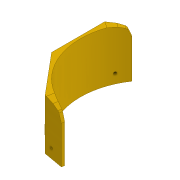
# Autodesk Inventor part: Delta Robot Siding Piece KUKA
Saved by Autodesk Inventor 2020 (Build 240168000, 168)
## iProperties
Created: 2021-04-12
Part Number: Delta Robot Siding Piece KUKA
Material: Generic
Document SubType Name: Modeling
Designer: Coy
Density: 1 g/cm^3
Appearance: Gold
Author: Coy
Autodesk Inventor part; units mm, degrees
ref_plane "YZ Plane" through (0, 0, 0) normal (1, 0, 0) x (0, 1, 0)
ref_plane "XZ Plane" through (0, 0, 0) normal (0, 1, 0) x (-1, 0, 0)
ref_plane "XY Plane" through (0, 0, 0) normal (0, 0, 1) x (1, 0, 0)
sketch "Sketch1" plane through (0, 0, 0) normal (0, 1, 0) x (-1, 0, 0)
  line L0 (68.675, -46.4884) -> (71.2969, -48.6885)
  line L1 (86.05, -31.1064) -> (71.2969, -48.6885)
  line L2 (86.05, 31.5329) -> (86.05, -31.1064)
  line L3 (45.7862, 79.5174) -> (86.05, 31.5329)
  line L4 (22.3355, 83.6524) -> (45.7862, 79.5174)
  line L5 (22.3355, 83.6524) -> (21.7555, 80.3631)
  arc A0 (68.675, -46.4884) -> (21.7555, 80.3631) centre (0, 0.2133) ccw
  constraints: 12 end point, 2 point on circle, 1 centre point
extrude "Extrusion1" add sketch "Sketch1" along normal blind 60
sketch "Sketch2" plane through (-86.05, 0, -31.1064) normal (-0.7660444, 0, -0.6427876) x (-0.6427876, 0, 0.7660444)
  circle A0 centre (-8.4518, 11) radius 1.625
  line L0 (-22.9518, 0) -> (0, 0) projected
  line L1 (-22.9518, 0) -> (-22.9518, 60) projected
  point P0 (-31.483, 0)
  dimension "d2" = 3.25
  dimension "d3" = 11
  dimension "d4" = 14.5
  constraints: 1 centre point
  measures "d2" diameter of A0
  measures "d3" distance from line of L0 A0.centre
  measures "d4" distance from line of L1 A0.centre
extrude "Extrusion2" cut sketch "Sketch2" against normal up to next
sketch "Sketch3" plane through (-22.3355, 0, 83.6524) normal (-0.1736482, 0, 0.9848078) x (0.9848078, 0, 0.1736482)
  circle A0 centre (-14.5, 11) radius 1.625
  line L0 (-23.8125, 0) -> (0, 0) projected
  line L1 (0, 0) -> (0, 60) projected
  point P0 (7.4701, 0)
  dimension "d7" = 3.25
  dimension "d8" = 11
  dimension "d9" = 14.5
  constraints: 1 centre point
  measures "d7" diameter of A0
  measures "d8" distance from line of L0 A0.centre
  measures "d9" distance from line of L1 A0.centre
extrude "Extrusion3" cut sketch "Sketch3" against normal up to next
chamfer "Chamfer5" distance 10 angle 45 2 edges at (-22.0455, 60, 82.0077) (-69.9859, 60, -47.5884)
chamfer "Chamfer6" distance 7 angle 45 2 edges at (-31.7611, 60, 79.5197) (-75.788, 60, -39.4028)
chamfer "Chamfer7" distance 5 angle 45 2 edges at (-38.4957, 60, 77.4021) (-79.5549, 60, -33.4258)
chamfer "Chamfer8" distance 5 angle 45 2 edges at (-22.0455, 50, 82.0077) (-69.9859, 50, -47.5884)
sketch "Sketch8" plane through (-86.05, 0, -31.1064) normal (-1, 0, 0) x (0, 0, 1)
  line L0 (0.07, 60.289) -> (62.7543, 60.289) construction
  line L1 (62.7543, 60.289) -> (62.7543, 0.051) construction
  line L2 (62.7543, 0.051) -> (0.07, 0.051) construction
  line L3 (0.07, 0.051) -> (0.07, 60.289) construction
  line L4 (35.582, 49.6056) -> (30.0412, 32.3549)
  line L5 (30.0412, 32.3549) -> (36.0961, 11.5056)
  line L6 (36.0961, 11.5056) -> (25.243, 11.5056)
  line L7 (25.243, 11.5056) -> (22.2156, 27.4425)
  line L8 (22.2156, 27.4425) -> (22.2156, 11.5056)
  line L9 (22.2156, 11.5056) -> (11.591, 11.5056)
  line L10 (11.591, 11.5056) -> (11.591, 49.6056)
  line L11 (11.591, 49.6056) -> (22.2156, 49.6056)
  line L12 (22.2156, 49.6056) -> (22.2156, 35.211)
  line L13 (22.2156, 35.211) -> (25.6429, 49.6056)
  line L14 (25.6429, 49.6056) -> (35.582, 49.6056)
  line L15 (60.2585, 49.6056) -> (60.2585, 24.3293)
  spline S0 degree 2 poles (60.2585, 24.3293) (60.2585, 20.0738) (59.6873, 16.4751) (56.8312, 12.6766) (52.2044, 10.7344) (49.0912, 10.7344) knots 0 0 0 1 2 3 4 4 4
  spline S1 degree 2 poles (49.0912, 10.7344) (45.664, 10.7344) (40.3517, 13.0193) (37.6955, 16.7607) (37.21, 20.8164) (37.21, 27.1568) knots 0 0 0 1 2 3 4 4 4
  line L16 (37.21, 27.1568) -> (37.21, 49.6056)
  line L17 (37.21, 49.6056) -> (47.8346, 49.6056)
  line L18 (47.8346, 49.6056) -> (47.8346, 21.3019)
  spline S2 degree 2 poles (47.8346, 21.3019) (47.8346, 18.9314) (48.2059, 17.9603) (48.6914, 17.9603) knots 0 0 0 1 2 2 2
  spline S3 degree 2 poles (48.6914, 17.9603) (49.234, 17.9603) (49.6339, 19.0742) (49.6339, 21.7589) knots 0 0 0 1 2 2 2
  line L19 (49.6339, 21.7589) -> (49.6339, 49.6056)
  line L20 (49.6339, 49.6056) -> (60.2585, 49.6056)
  point P0 (31.1064, 0)
  constraints: 2 other
extrude "Extrusion8" add sketch "Sketch8" along normal blind 1.27
sketch "Sketch9" plane through (-45.7862, 0, 79.5174) normal (-0.7660444, 0, 0.6427876) x (0.6427876, 0, 0.7660444)
  line L0 (-62.4698, 60.3336) -> (-0.1509, 60.3336) construction
  line L1 (-0.1509, 60.3336) -> (-0.1509, -0.0863) construction
  line L2 (-0.1509, -0.0863) -> (-62.4698, -0.0863) construction
  line L3 (-62.4698, -0.0863) -> (-62.4698, 60.3336) construction
  line L4 (-36.5367, 49.1737) -> (-42.0775, 31.923)
  line L5 (-42.0775, 31.923) -> (-36.0226, 11.0737)
  line L6 (-36.0226, 11.0737) -> (-46.8757, 11.0737)
  line L7 (-46.8757, 11.0737) -> (-49.9031, 27.0105)
  line L8 (-49.9031, 27.0105) -> (-49.9031, 11.0737)
  line L9 (-49.9031, 11.0737) -> (-60.5277, 11.0737)
  line L10 (-60.5277, 11.0737) -> (-60.5277, 49.1737)
  line L11 (-60.5277, 49.1737) -> (-49.9031, 49.1737)
  line L12 (-49.9031, 49.1737) -> (-49.9031, 34.7791)
  line L13 (-49.9031, 34.7791) -> (-46.4758, 49.1737)
  line L14 (-46.4758, 49.1737) -> (-36.5367, 49.1737)
  line L15 (-17.2011, 49.1737) -> (-11.5746, 11.0737)
  line L16 (-11.5746, 11.0737) -> (-22.4277, 11.0737)
  line L17 (-22.4277, 11.0737) -> (-22.9418, 17.7569)
  line L18 (-22.9418, 17.7569) -> (-25.4837, 17.7569)
  line L19 (-25.4837, 17.7569) -> (-26.0549, 11.0737)
  line L20 (-26.0549, 11.0737) -> (-36.9651, 11.0737)
  line L21 (-36.9651, 11.0737) -> (-31.9955, 49.1737)
  line L22 (-31.9955, 49.1737) -> (-17.2011, 49.1737)
  spline S0 degree 2 poles (-23.2274, 25.2969) (-23.9128, 31.0376) (-24.3127, 39.9486) knots 0 0 0 1 1 1
  spline S1 degree 2 poles (-24.3127, 39.9486) (-25.1695, 29.6667) (-25.5122, 25.2969) knots 0 0 0 1 1 1
  line L23 (-25.5122, 25.2969) -> (-23.2274, 25.2969)
  point P0 (-31.483, 0)
  constraints: 2 other
extrude "Extrusion9" add sketch "Sketch9" along normal blind 1.27
chamfer "Chamfer10" distance 1 angle 45 14 edges at (-86.05, 11.5056, -14.2031) (-86.05, 11.5056, -0.4368) (-86.05, 49.6056, -14.2031) (-86.05, 49.6056, -0.4939) (-86.05, 49.6056, 11.4159) (-86.05, 49.6056, 23.8398) (-81.278, 11.0737, 37.2199) (-69.2257, 11.0737, 51.5833) (-56.7144, 11.0737, 66.4937) (-61.3499, 17.7569, 60.9693) (-61.4509, 25.2969, 60.849) (-72.466, 49.1737, 47.7217) (-81.278, 49.1737, 37.2199) (-61.5977, 49.1737, 60.674)
body "Solid1"
